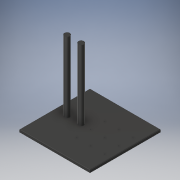
# Autodesk Inventor part: FTK100
Saved by Autodesk Inventor 2019.4 (Build 234330000, 330)
## iProperties
Created: 2021-01-23
Part Number: FTK100
Material: UHMW, Black
Document SubType Name: Modeling
Designer: caleb
Density: 0.94 g/cm^3
Appearance: Smooth - Black
Author: caleb
Autodesk Inventor part; units mm, degrees
ref_plane "YZ Plane" through (0, 0, 0) normal (1, 0, 0) x (0, 1, 0)
ref_plane "XZ Plane" through (0, 0, 0) normal (0, 1, 0) x (-1, 0, 0)
ref_plane "XY Plane" through (0, 0, 0) normal (0, 0, 1) x (1, 0, 0)
sketch "Sketch1" plane through (0, 0, 0) normal (0, 1, 0) x (-1, 0, 0)
  line L0 (-127, 127) -> (127, 127)
  line L1 (127, 127) -> (127, -127)
  line L2 (127, -127) -> (-127, -127)
  line L3 (-127, -127) -> (-127, 127)
  line L4 (-127, 127) -> (127, -127) construction
  line L5 (127, 127) -> (-127, -127) construction
  circle A0 centre (31.75, 0) radius 9.525
  circle A1 centre (82.55, 0) radius 9.525
  point P0 (0, 0)
  point P1 (-104.775, 50.8)
  point P2 (-53.975, 50.8)
  point P3 (-3.175, 50.8)
  point P4 (-104.775, 0)
  point P5 (-53.975, 0)
  point P6 (-3.175, 0)
  point P7 (-104.775, -50.8)
  point P8 (-53.975, -50.8)
  point P9 (-3.175, -50.8)
  dimension "d0" = 254
  dimension "d1" = 254
  dimension "d2" = 76.2
  dimension "d3" = 22.225
  dimension "d6" = 50.8
  dimension "d9" = 50.8
  dimension "d12" = 19.05
  dimension "d13" = 158.75
  dimension "d14" = 19.05
  dimension "d15" = 50.8
  constraints: 12 end point, 2 centre point, 2 horizontal, 2 midpoint, 2 parallel, 1 perpendicular, 1 vertical, 8 other
  measures "d0" distance of L0.end L1.end
  measures "d1" distance of L1.end L2.end
  measures "d2" distance from line of L0 point (-104.775, 50.8)
  measures "d3" distance from line of L3 point (-104.775, 50.8)
  measures "d6" distance of point (-104.775, 50.8) point (-53.975, 50.8)
  measures "d9" distance of point (-104.775, 50.8) point (-104.775, 0)
  measures "d12" diameter of A0
  measures "d13" distance from line of L3 A0.centre
  measures "d14" diameter of A1
  measures "d15" distance of A1.centre A0.centre
extrude "Extrusion1" add sketch "Sketch1" against normal blind 9.525 contours L0 L1 L2 L3 | A0 | A1
extrude "Extrusion2" add sketch "Sketch1" along normal blind 254 contours A0 | A1
hole "Hole1" at (104.775, 0, 50.8) at (53.975, 0, 50.8) at (3.175, 0, 50.8) at (104.775, 0, 0) at (53.975, 0, 0) at (3.175, 0, 0) at (104.775, 0, -50.8) at (53.975, 0, -50.8) at (3.175, 0, -50.8) direction (0, -1, 0) diameter 3.9624 end through all thread size "10-32 UNF" class "2B" standard "ANSI Unified Screw Threads"
chamfer "Chamfer1" distance 1.5875 angle 45 4 edges at (0, 0, 127) (127, 0, 0) (0, 0, -127) (-127, 0, 0)
body "Solid1"
